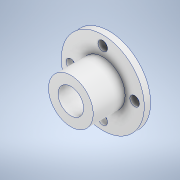
# Autodesk Inventor part: AcopleBrida8mm
Saved by Autodesk Inventor 2021 (Build 250183000, 183)
## iProperties
Created: 2022-10-28
Part Number: AcopleBrida8mm
Material: Aluminio 6061
Document SubType Name: Modeling
Designer: zulet
Density: 2.7 g/cm^3
Appearance: Aluminio - Plano
Mass: 5.24206 g
Surface Area: 18.8496 cm^2
Volume: 1.9415 cm^3
Author: zulet
Autodesk Inventor part; units mm, degrees
ref_plane "YZ Plane" through (0, 0, 0) normal (1, 0, 0) x (0, 1, 0)
ref_plane "Work Plane1" through (0, 0, 0) normal (0, 0, 1) x (1, 0, 0)
sketch "Sketch1" plane through (0, 0, 0) normal (0, 0, 1) x (1, 0, 0)
  circle A0 centre (0, -92.5) radius 4 projected
  circle A1 centre (0, -102.5) radius 1.5 projected
  circle A2 centre (-10, -92.5) radius 1.5 projected
  circle A3 centre (0, -82.5) radius 1.5 projected
  circle A4 centre (10, -92.5) radius 1.5 projected
  circle A5 centre (0, -92.5) radius 13
  circle A6 centre (0, -92.5) radius 7
  point P0 (0, 0)
  dimension "d0" = 26
  dimension "d1" = 14
  constraints: 2 centre point, 2 coincident
  measures "d0" diameter of A5
  measures "d1" diameter of A6
extrude "Extrusion1" add sketch "Sketch1" along normal blind 2 contours A5
ref_plane "Work Plane2" through (0, 0, 0) normal (0, 0, 1) x (1, 0, 0)
sketch "Sketch2" plane through (0, 0, 0) normal (0, 0, 1) x (1, 0, 0)
  circle A0 centre (0, -92.5) radius 7 projected
  circle A1 centre (0, -92.5) radius 4 projected
  point P0 (0, 0)
extrude "Extrusion2" add sketch "Sketch2" along normal blind 12
body "Solid1"
